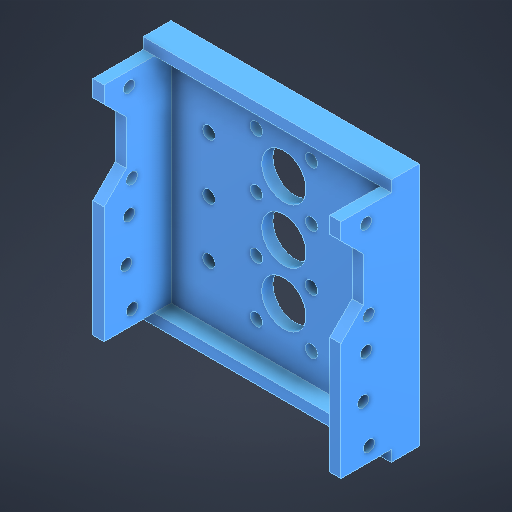
# Autodesk Inventor part: 3 Cilindros
Saved by Autodesk Inventor 2027 (Build 310192060, 192F)
## iProperties
Created: 2019-01-24
Part Number: 3 Cilindros
Material: Genérico
Description: STEP AP214
Document SubType Name: Modeling
Designer: paulo
Density: 1 g/cm^3
Appearance: Padrão
Sending System: SolidWorks 2018
Preprocessor: SwSTEP 2.0
Title: ²à¸Ç.STEP
Revision Number: ÈÎºÎ
Autodesk Inventor part; units mm, degrees
ref_plane "YZ Plane" through (0, 0, 0) normal (1, 0, 0) x (0, 1, 0)
ref_plane "Plano de trabalho1" through (20.3, 41, 0) normal (0, 0, -1) x (-1, 0, 0)
sketch "Esboço2" plane through (20.3, 41, 0) normal (0, 0, -1) x (-1, 0, 0)
  line L0 (-1, 1) -> (0, 0) projected
  line L1 (0, -40) -> (40.6, -40) projected
  line L2 (0, 0) -> (40.6, 0)
  line L3 (40.6, 0) -> (40.6, -40)
  line L4 (40.6, -40) -> (0, -40)
  line L5 (0, -40) -> (0, 0)
  circle A0 centre (20.3, -20) radius 4 projected
  circle A1 centre (20.3, -20) radius 4
  circle A2 centre (20.3, -10.1005) radius 4 projected
  circle A3 centre (20.3, -10.1005) radius 4
  circle A4 centre (20.3, -29.8995) radius 4 projected
  circle A5 centre (20.3, -29.8995) radius 4
  circle A6 centre (25.2497, -5.1508) radius 1.1 projected
  circle A7 centre (25.2497, -5.1508) radius 1.1
  circle A8 centre (25.2497, -15.0503) radius 1.1 projected
  circle A9 centre (25.2497, -15.0503) radius 1.1
  circle A10 centre (25.2497, -24.9497) radius 1.1 projected
  circle A11 centre (25.2497, -24.9497) radius 1.1
  circle A12 centre (25.2497, -34.8492) radius 1.1 projected
  circle A13 centre (25.2497, -34.8492) radius 1.1
  circle A14 centre (33.8, -10) radius 1.1 projected
  circle A15 centre (33.8, -10) radius 1.1
  circle A16 centre (33.8, -30) radius 1.1 projected
  circle A17 centre (33.8, -30) radius 1.1
  circle A18 centre (33.8, -20) radius 1.1 projected
  circle A19 centre (33.8, -20) radius 1.1
  circle A20 centre (15.3503, -5.1508) radius 1.1 projected
  circle A21 centre (15.3503, -5.1508) radius 1.1
  circle A22 centre (15.3503, -15.0503) radius 1.1 projected
  circle A23 centre (15.3503, -15.0503) radius 1.1
  circle A24 centre (15.3503, -24.9497) radius 1.1 projected
  circle A25 centre (15.3503, -24.9497) radius 1.1
  circle A26 centre (15.3503, -34.8492) radius 1.1 projected
  circle A27 centre (15.3503, -34.8492) radius 1.1
  circle A28 centre (6.8, -10) radius 1.1 projected
  circle A29 centre (6.8, -10) radius 1.1
  circle A30 centre (6.8, -20) radius 1.1 projected
  circle A31 centre (6.8, -20) radius 1.1
  circle A32 centre (6.8, -30) radius 1.1 projected
  circle A33 centre (6.8, -30) radius 1.1
  line L6 (-1, 1) -> (41.6, 1)
  line L7 (41.6, 1) -> (41.6, -41)
  line L8 (41.6, -41) -> (-1, -41)
  line L9 (-1, -41) -> (-1, 1)
  line L10 (-1, 1) -> (41.6, -41) construction
  line L11 (41.6, 1) -> (-1, -41) construction
  line L12 (66.6981, -6.0879) -> (67.6981, -7.0879)
  line L13 (67.6981, -47.0879) -> (108.2981, -47.0879)
  line L14 (67.6981, -7.0879) -> (108.2981, -7.0879)
  line L15 (108.2981, -7.0879) -> (108.2981, -47.0879)
  line L16 (108.2981, -47.0879) -> (67.6981, -47.0879)
  line L17 (67.6981, -47.0879) -> (67.6981, -7.0879)
  circle A34 centre (87.9981, -27.0879) radius 4
  circle A35 centre (87.9981, -27.0879) radius 4
  circle A36 centre (87.9981, -17.1884) radius 4
  circle A37 centre (87.9981, -17.1884) radius 4
  circle A38 centre (87.9981, -36.9874) radius 4
  circle A39 centre (87.9981, -36.9874) radius 4
  circle A40 centre (92.9478, -12.2387) radius 1.1
  circle A41 centre (92.9478, -12.2387) radius 1.1
  circle A42 centre (92.9478, -22.1382) radius 1.1
  circle A43 centre (92.9478, -22.1382) radius 1.1
  circle A44 centre (92.9478, -32.0377) radius 1.1
  circle A45 centre (92.9478, -32.0377) radius 1.1
  circle A46 centre (92.9478, -41.9372) radius 1.1
  circle A47 centre (92.9478, -41.9372) radius 1.1
  circle A48 centre (101.4981, -17.0879) radius 1.1
  circle A49 centre (101.4981, -17.0879) radius 1.1
  circle A50 centre (101.4981, -37.0879) radius 1.1
  circle A51 centre (101.4981, -37.0879) radius 1.1
  circle A52 centre (101.4981, -27.0879) radius 1.1
  circle A53 centre (101.4981, -27.0879) radius 1.1
  circle A54 centre (83.0483, -12.2387) radius 1.1
  circle A55 centre (83.0483, -12.2387) radius 1.1
  circle A56 centre (83.0483, -22.1382) radius 1.1
  circle A57 centre (83.0483, -22.1382) radius 1.1
  circle A58 centre (83.0483, -32.0377) radius 1.1
  circle A59 centre (83.0483, -32.0377) radius 1.1
  circle A60 centre (83.0483, -41.9372) radius 1.1
  circle A61 centre (83.0483, -41.9372) radius 1.1
  circle A62 centre (74.4981, -17.0879) radius 1.1
  circle A63 centre (74.4981, -17.0879) radius 1.1
  circle A64 centre (74.4981, -27.0879) radius 1.1
  circle A65 centre (74.4981, -27.0879) radius 1.1
  circle A66 centre (74.4981, -37.0879) radius 1.1
  circle A67 centre (74.4981, -37.0879) radius 1.1
  line L18 (66.6981, -6.0879) -> (109.2981, -48.0879) construction
  line L19 (109.2981, -6.0879) -> (66.6981, -48.0879) construction
  line L20 (67.6981, -7.0879) -> (65.6981, -7.0879)
  line L21 (108.2981, -7.0879) -> (110.2981, -7.0879)
  line L22 (108.2981, -47.0879) -> (110.2981, -47.0879)
  line L23 (67.6981, -47.0879) -> (65.6981, -47.0879)
  line L24 (65.6981, -49.0879) -> (110.2981, -49.0879)
  line L25 (110.2981, -49.0879) -> (110.2981, -5.0879)
  line L26 (110.2981, -5.0879) -> (65.6981, -5.0879)
  line L27 (65.6981, -5.0879) -> (65.6981, -49.0879)
  line L28 (65.6981, -49.0879) -> (110.2981, -5.0879) construction
  line L29 (110.2981, -49.0879) -> (65.6981, -5.0879) construction
  point P0 (20.3, -41)
  point P1 (87.9981, -48.0879)
  dimension "d2" = 44.6
  dimension "d3" = 44
  constraints: 56 end point, 51 centre point, 34 coincident, 8 parallel, 6 midpoint, 6 perpendicular, 5 horizontal, 5 point on line
  measures "d2" distance of L26.end L25.end
  measures "d3" distance of L25.end L24.end
extrude "Extrusão1" add sketch "Esboço2" against normal blind 2 contours L17 L14 L15 L13
extrude "Extrusão2" add sketch "Esboço2" against normal blind 5 contours L13 L22 L25 L24 L27 L23 | L20 L27 L26 L25 L21 L14
extrude "Extrusão3" add sketch "Esboço2" against normal blind 14.04 contours L23 L27 L20 L17 | L15 L21 L25 L22
ref_plane "Plano de trabalho4" through (-89.9981, -8.0879, 0) normal (-1, 0, 0) x (0, 0, 1)
sketch "Esboço6" plane through (-89.9981, -8.0879, 0) normal (-1, 0, 0) x (0, 0, 1)
  circle A0 centre (9.54, 39.48) radius 1
  circle A1 centre (9.04, 25) radius 1
  circle A2 centre (9.54, 19.5) radius 1
  circle A3 centre (9, 4.5879) radius 1
  circle A4 centre (10.04, 12) radius 1
  line L0 (14.04, 35) -> (14.04, 42)
  line L1 (10.04, 35) -> (10.04, 27)
  line L2 (10.04, 35) -> (14.04, 39)
  line L3 (10.04, 27) -> (14.04, 23)
  line L4 (14.04, 39) -> (14.04, 23)
  line L5 (14.04, 42) -> (14.04, 2) projected
  point P0 (0, 8.0879)
  dimension "d12" = 2
  dimension "d14" = 2
  dimension "d17" = 2
  dimension "d19" = 2
  dimension "d21" = 2
  dimension "d24" = 4
  dimension "d26" = 8
  constraints: 10 end point, 5 centre point, 2 point on line, 1 collinear, 1 vertical
  measures "d12" diameter of A0
  measures "d14" diameter of A1
  measures "d17" diameter of A2
  measures "d19" diameter of A3
  measures "d21" diameter of A4
  measures "d24" distance of L0.start L1.start
  measures "d26" distance of L1.start L1.end
extrude "Extrusão4" cut sketch "Esboço6" against normal blind 50 contours A0 | A1 | A2 | A3 | A4
extrude "Extrusão5" cut sketch "Esboço6" against normal blind 50 contours L4 L3 L1 L2 L0
